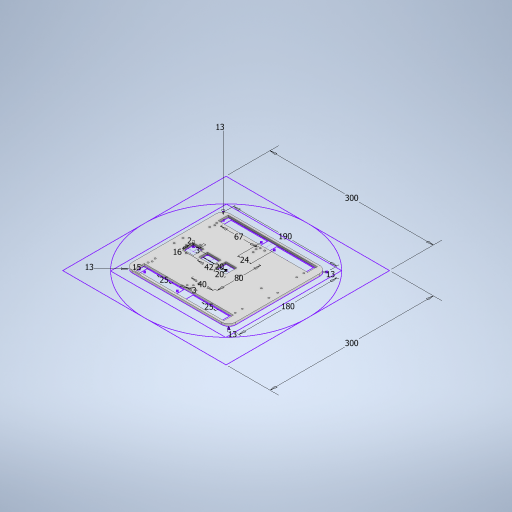
# Autodesk Inventor part: основа
Saved by Autodesk Inventor 2023 (Build 270158000, 158)
## iProperties
Created: 2025-12-12
Part Number: основа
Material: Типовые
Document SubType Name: Modeling
Designer: garin
Density: 1 g/cm^3
Appearance: По умолчанию
Author: garin
Autodesk Inventor part; units mm, degrees
ref_plane "YZ Plane" through (0, 0, 0) normal (1, 0, 0) x (0, 1, 0)
ref_plane "XZ Plane" through (0, 0, 0) normal (0, 1, 0) x (-1, 0, 0)
ref_plane "XY Plane" through (0, 0, 0) normal (0, 0, 1) x (1, 0, 0)
sketch "Эскиз1" plane through (0, 0, 0) normal (0, 1, 0) x (-1, 0, 0)
  line L0 (150, 150) -> (-150, 150)
  line L1 (-150, 150) -> (-150, -150)
  line L2 (-150, -150) -> (150, -150)
  line L3 (150, -150) -> (150, 150)
  circle A0 centre (0, 0) radius 150
  line L4 (-106, -106) -> (105.4385, -106)
  line L5 (105.4385, -106) -> (105.4385, 106.6899)
  line L6 (105.4385, 106.6899) -> (-106, 106.6899)
  line L7 (-106, 106.6899) -> (-106, -106)
  line L8 (82, 90) -> (-80, 90)
  line L9 (-95, 75) -> (-95, -75)
  line L10 (-80, -90) -> (82, -90)
  line L11 (95, -77) -> (95, 77)
  arc A1 (95, 77) -> (82, 90) centre (82, 77) ccw
  arc A2 (82, -90) -> (95, -77) centre (82, -77) ccw
  line L12 (72, 84.5) -> (12, 84.5)
  line L13 (12, 69.5) -> (72, 69.5)
  line L14 (-80, 90) -> (-82, 90)
  line L15 (-95, 77) -> (-95, 75)
  arc A3 (-82, 90) -> (-95, 77) centre (-82, 77) ccw
  line L16 (-80, -90) -> (-82, -90)
  line L17 (-95, -77) -> (-95, -75)
  arc A4 (-95, -77) -> (-82, -90) centre (-82, -77) ccw
  line L18 (76.9408, 68) -> (82, 68)
  line L19 (82, 68) -> (-82, 68)
  line L20 (-82, 86) -> (82, 86)
  line L21 (82, -68) -> (-82, -68)
  line L22 (-82, -68) -> (-82, -86)
  line L23 (-82, -86) -> (82, -86)
  line L24 (-82, 68) -> (-72, 68)
  line L25 (-72, 86) -> (-82, 86)
  line L26 (-82, 86) -> (-82, 68)
  line L27 (-82, -86) -> (-72, -86)
  line L28 (-72, -68) -> (-82, -68)
  line L29 (-82, -68) -> (-82, -86)
  line L30 (82, -86) -> (72, -86)
  line L31 (72, -68) -> (82, -68)
  line L32 (82, -68) -> (82, -86)
  line L33 (72, 68) -> (82, 68)
  line L34 (82, 68) -> (82, 86)
  line L35 (82, 86) -> (72, 86)
  line L36 (42, 68) -> (54.5, 68)
  line L37 (42, 8) -> (17, 8)
  line L38 (29.5, 8) -> (29.5, 68)
  line L39 (29.5, 68) -> (54.5, 68)
  line L40 (54.5, 68) -> (54.5, 8)
  line L41 (42, -8) -> (17, -8)
  line L42 (29.5, -8) -> (29.5, -68)
  line L43 (29.5, -68) -> (54.5, -68)
  line L44 (54.5, -68) -> (54.5, -8)
  line L45 (-42, 68) -> (-29.5, 68)
  line L46 (-54.5, 8) -> (-54.5, 68)
  line L47 (-54.5, 68) -> (-29.5, 68)
  line L48 (-29.5, 68) -> (-29.5, 8)
  line L49 (-54.5, -8) -> (-54.5, -68)
  line L50 (-54.5, -68) -> (-29.5, -68)
  line L51 (-29.5, -68) -> (-29.5, -8)
  line L52 (75.5, -84.5) -> (8.5, -84.5)
  line L53 (8.5, -84.5) -> (8.5, -69.5)
  line L54 (8.5, -69.5) -> (75.5, -69.5)
  line L55 (75.5, -69.5) -> (75.5, -84.5)
  line L56 (0, -86) -> (0, -44.6693) construction
  line L57 (-75.5, -84.5) -> (-8.5, -84.5)
  line L58 (-8.5, -84.5) -> (-8.5, -69.5)
  line L59 (-8.5, -69.5) -> (-75.5, -69.5)
  line L60 (-75.5, -69.5) -> (-75.5, -84.5)
  line L61 (75.5, 84.5) -> (8.5, 84.5)
  line L62 (8.5, 84.5) -> (8.5, 69.5)
  line L63 (8.5, 69.5) -> (75.5, 69.5)
  line L64 (75.5, 69.5) -> (75.5, 84.5)
  line L65 (-8.5, 84.5) -> (-8.5, 69.5)
  line L66 (-8.5, 69.5) -> (-75.5, 69.5)
  line L67 (-75.5, 69.5) -> (-75.5, 84.5)
  line L68 (-75.5, 84.5) -> (-8.5, 84.5)
  line L69 (54.5, 8) -> (29.5, 8)
  line L70 (17, 8) -> (17, -8)
  line L71 (29.5, -8) -> (54.5, -8)
  line L72 (42, -8) -> (42, 8)
  line L73 (-54.5, 8) -> (-54.5, -8)
  line L74 (-29.5, -8) -> (-29.5, 8)
  line L75 (20, -40) -> (-20, -40)
  line L76 (-20, -40) -> (-20, 40)
  line L77 (-20, 40) -> (20, 40)
  line L78 (20, 40) -> (20, -40)
  line L79 (20, 25) -> (20, 40)
  line L80 (20, 30) -> (20, 40)
  line L81 (-10, -10) -> (10, -10)
  line L82 (10, -10) -> (10, 10)
  line L83 (10, 10) -> (-10, 10)
  line L84 (-10, 10) -> (-10, -10)
  point P0 (-95, -90)
  point P1 (-95, 90)
  point P2 (95, -90)
  point P3 (-12, -77)
  point P4 (12, -77)
  point P5 (12, 77)
  point P6 (72, 77)
  point P7 (42, 8)
  point P8 (42, -8)
  point P9 (-42, -69.5)
  point P10 (42, -8)
  point P11 (-9, 0)
  point P12 (42, 0)
  point P13 (29.5, 0)
  dimension "d2" = 300
  dimension "d3" = 300
  dimension "d8" = 190
  dimension "d9" = 180
  dimension "d10" = 13
  dimension "d11" = 13
  dimension "d31" = 13
  dimension "d32" = 13
  dimension "d41" = 15
  dimension "d42" = 24
  dimension "d47" = 25
  dimension "d51" = 25
  dimension "d52" = 16
  dimension "d112" = 67
  dimension "d123" = 40
  dimension "d124" = 80
  dimension "d147" = 20
  dimension "d148" = 20
  constraints: 170 end point, 28 parallel, 20 horizontal, 16 point on line, 13 perpendicular, 8 point on circle, 8 tangent, 4 centre point, 4 symmetric about line, 1 coincident, 1 midpoint, 1 vertical, 3 other
  measures "d2" distance of L2.end L1.end
  measures "d3" distance of L1.end L0.end
  measures "d8" distance of point (95, -90) point (-95, -90)
  measures "d9" distance of point (-95, -90) point (-95, 90)
  measures "d10" radius of A1
  measures "d11" radius of A2
  measures "d31" radius of A3
  measures "d32" radius of A4
  measures "d41" distance of L12.start L13.end
  measures "d42" distance of point (-12, -77) point (12, -77)
  measures "d47" distance of L38.end L39.end
  measures "d51" distance of L46.end L47.end
  measures "d52" distance of point (42, 8) point (42, -8)
  measures "d112" distance of L53.end L54.end
  measures "d123" distance of L76.end L77.end
  measures "d124" distance of L75.end L76.end
  measures "d147" distance of L83.end L82.end
  measures "d148" distance of L82.end L81.end
extrude "Выдавливание1" add sketch "Эскиз1" along normal blind 4 contours A1 L11 A2 L10 L16 A4 L17 L9 L15 A3 L14 L8 | L40 L69 L37 L38 L19 | L38 L37 L78 L77 L76 L75 L41 L42 L21 L51 L74 L48 L19 | L72 L41 L78 L37 | L48 L74 L51 L21 L49 L73 L46 L19 | L71 L44 L21 L42 L41 | L78 L41 L70 L37 | L37 L70 L41 L78 L75 L76 L77 | L84 L83 L82 L81
sketch "Эскиз2" plane through (0, 0, 0) normal (0, -1, 0) x (1, 0, 0)
  line L0 (-82, -68) -> (-82, -86) projected
  line L1 (-95, -77) -> (-95, 77) projected
  line L2 (-95, -68) -> (-95, -56.3368)
  line L3 (-95, -45) -> (-95, -68) construction
  line L4 (-95, -68) -> (-80, -68) construction
  line L5 (-95, -63) -> (-95, -68)
  line L6 (-95, -50) -> (-95, -45)
  circle A0 centre (-80, -63) radius 1.5
  circle A1 centre (-80, -50) radius 1.5
  line L7 (95, 77) -> (95, -77) projected
  line L8 (95, -68) -> (95, -45)
  line L9 (-95, -45) -> (-95, -68)
  line L10 (82, -90) -> (-82, -90) projected
  circle A2 centre (80, -63) radius 1.5
  circle A3 centre (80, -50) radius 1.5
  line L11 (-95, -68) -> (-95, -63)
  line L12 (95, -63) -> (95, -68)
  line L13 (95, -45) -> (95, -50)
  line L14 (-95, -50) -> (-95, -45)
  circle A4 centre (0, -50) radius 1.5
  circle A5 centre (0, -63) radius 1.5
  line L15 (-95, 0) -> (95, 0)
  circle A6 centre (-80, 63) radius 1.5
  circle A7 centre (-80, 50) radius 1.5
  circle A8 centre (80, 63) radius 1.5
  circle A9 centre (80, 50) radius 1.5
  circle A10 centre (0, 50) radius 1.5
  circle A11 centre (0, 63) radius 1.5
  line L16 (-95, -68) -> (95, -68)
  line L17 (95, -68) -> (95, -45)
  line L18 (95, -45) -> (-95, -45)
  line L19 (-95, -45) -> (-95, -68)
  line L20 (-82, 68) -> (-95, 68)
  line L21 (-95, 68) -> (95, 68)
  line L22 (95, 68) -> (95, 45)
  line L23 (95, 45) -> (-95, 45)
  line L24 (-95, 45) -> (-95, 68)
  point P0 (0, 0)
  dimension "d64" = 23
  constraints: 42 end point, 12 centre point, 7 parallel, 6 symmetric about line, 5 point on line, 3 horizontal, 3 perpendicular, 2 midpoint, 6 other
  measures "d64" distance of L21.end L22.end
extrude "Выдавливание2" cut sketch "Эскиз2" against normal blind 4 contours A0 | A1 | A2 | A3 | A4 | A5 | A6 | A7 | A8 | A9 | A10 | A11
sketch "Эскиз3" plane through (0, 0, 0) normal (0, -1, 0) x (1, 0, 0)
  line L0 (-95, -77) -> (-95, 77) projected
  line L1 (-95, 10) -> (-95, 0)
  circle A0 centre (-73, 0) radius 1.5
  circle A1 centre (-60, -13) radius 1.5
  circle A2 centre (-60, 13) radius 1.5
  line L2 (-70, -10) -> (-80, -10)
  line L3 (-60, -10) -> (-80, -10)
  line L4 (-50, -10) -> (-68, -10)
  line L5 (-70, -8) -> (-70, 8)
  line L6 (-68, 10) -> (-50, 10)
  line L7 (-50, 10) -> (-50, -10)
  arc A3 (-70, -8) -> (-68, -10) centre (-68, -8) ccw
  arc A4 (-68, 10) -> (-70, 8) centre (-68, 8) ccw
  line L8 (0, 0) -> (-42, 0)
  line L9 (-42, 0) -> (-42, 8)
  line L10 (-42, 8) -> (0, 8)
  line L11 (0, 8) -> (0, 0)
  point P0 (-70, -13)
  point P1 (-78, -10)
  point P2 (-70, 0)
  point P3 (-60, 0)
  dimension "d79" = 3
  dimension "d87" = 2
  dimension "d149" = 42
  constraints: 22 end point, 5 centre point, 4 parallel, 4 point on circle, 4 tangent, 3 horizontal, 2 perpendicular, 1 coincident, 1 equal radius, 1 midpoint
  measures "d79" diameter of A1
  measures "d87" radius of A3
  measures "d149" distance of L9.end L10.end
extrude "Выдавливание3" cut sketch "Эскиз3" against normal blind 4 contours A0 | A1 | A2
extrude "Выдавливание4" cut sketch "Эскиз3" against normal blind 4 contours L3 A3 L5 A4 L6 L7 L4
sketch "Эскиз4" plane through (0, 0, 0) normal (0, -1, 0) x (1, 0, 0)
  circle A0 centre (-80, 63) radius 1.5 projected
  circle A1 centre (-78, 57.5) radius 1.5
  circle A2 centre (0, 63) radius 1.5 projected
  circle A3 centre (-2.2, 57.5) radius 1.5
  line L0 (-47.745, 0) -> (17.0058, 0) construction
  circle A4 centre (-78, -57.5) radius 1.5
  circle A5 centre (-2.2, -57.5) radius 1.5
  point P0 (0, 0)
  dimension "d92" = 3
  dimension "d95" = 3
  constraints: 4 centre point, 2 end point, 2 symmetric about line, 1 horizontal, 2 other
  measures "d92" diameter of A1
  measures "d95" diameter of A3
extrude "Выдавливание5" cut sketch "Эскиз4" against normal blind 4 contours A1 | A3 | A4 | A5
sketch "Эскиз5" plane through (0, 0, 0) normal (0, -1, 0) x (1, 0, 0)
  line L0 (82, -68) -> (-82, -68) projected
  line L1 (-82, -86) -> (82, -86) projected
  line L2 (-90.0897, 0) -> (-46.8311, 0) construction
  line L3 (0, -13.4429) -> (0, 16.6684) construction
  circle A0 centre (-87, -8.1) radius 1.5
  line L4 (-82, 68) -> (82, 68) construction
  line L5 (0, 68) -> (-4.5, 68) construction
  line L6 (-4.5, 63) -> (0, 63) construction
  line L7 (0, 63) -> (0, 68) construction
  line L8 (-17.2785, 0) -> (16.6341, 0) construction
  circle A1 centre (-8.1, 63) radius 1.5
  circle A2 centre (-87, 8.1) radius 1.5
  circle A3 centre (87, -8.1) radius 1.5
  circle A4 centre (87, 8.1) radius 1.5
  circle A5 centre (8.1, 63) radius 1.5
  circle A6 centre (-8.1, -63) radius 1.5
  circle A7 centre (8.1, -63) radius 1.5
  point P0 (0, 0)
  point P1 (-87, 0)
  dimension "d115" = 3
  constraints: 12 end point, 8 centre point, 6 symmetric about line, 3 horizontal, 1 midpoint, 1 parallel, 1 vertical, 6 other
  measures "d115" diameter of A1
extrude "Выдавливание6" cut sketch "Эскиз5" against normal blind 4 contours A0
extrude "Выдавливание7" cut sketch "Эскиз5" against normal blind 4 contours A1
extrude "Выдавливание8" cut sketch "Эскиз1" along normal blind 4 contours L72 L41 L78 L37 | L78 L41 L70 L37
extrude "Выдавливание9" cut sketch "Эскиз1" along normal blind 4 contours L84 L83 L82 L81
sketch "Эскиз6" plane through (0, 4, 0) normal (0, 1, 0) x (1, 0, 0)
  line L0 (15, -37.5) -> (75, -37.5)
  line L1 (75, -37.5) -> (75, 37.5)
  line L2 (75, 37.5) -> (15, 37.5)
  line L3 (15, 37.5) -> (15, -37.5)
  line L4 (15, -37.5) -> (25, -37.5)
  line L5 (45, -37.5) -> (45, 37.5) construction
  circle A0 centre (25, 0) radius 1.5
  circle A1 centre (65, 0) radius 1.5
  point P0 (0, 0)
  dimension "d139" = 60
  dimension "d140" = 75
  dimension "d141" = 10
  dimension "d142" = 3
  constraints: 12 end point, 2 centre point, 2 midpoint, 2 parallel, 1 coincident, 1 horizontal, 1 perpendicular, 1 point on line, 1 symmetric about line, 1 other
  measures "d139" distance of L2.end L1.end
  measures "d140" distance of L1.end L0.end
  measures "d141" distance of L0.start L4.end
  measures "d142" diameter of A0
extrude "Выдавливание10" cut sketch "Эскиз6" against normal blind 4 contours A0 | A1
extrude "Выдавливание11" cut sketch "Эскиз5" against normal blind 10 contours A2
extrude "Выдавливание12" cut sketch "Эскиз5" against normal blind 10 contours A3 | A4 | A5 | A6 | A7
